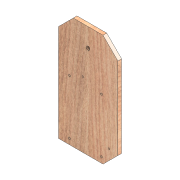
# Autodesk Inventor part: legno
Saved by Autodesk Inventor 2022 (Build 260153000, 153)
## iProperties
Created: 2025-08-06
Part Number: legno
Material: Wood (Birch)
Document SubType Name: Modeling
Designer: sacchie
Density: 0.55 g/cm^3
Appearance: Birch - Natural Polished
Author: sacchie
Autodesk Inventor part; units mm, degrees
ref_plane "YZ Plane" through (0, 0, 0) normal (1, 0, 0) x (0, 1, 0)
ref_plane "XZ Plane" through (0, 0, 0) normal (0, 1, 0) x (-1, 0, 0)
ref_plane "XY Plane" through (0, 0, 0) normal (0, 0, 1) x (1, 0, 0)
sketch "Sketch1" plane through (0, 0, 0) normal (0, 0, 1) x (1, 0, 0)
  line L0 (0, 0) -> (-160, 0)
  line L1 (-160, 0) -> (-160, 300)
  line L2 (-160, 300) -> (0, 300)
  line L3 (0, 300) -> (0, 0)
  dimension "d0" = 160
  dimension "d1" = 300
  constraints: 8 end point, 2 parallel, 1 horizontal, 1 perpendicular
  measures "d0" distance of L1.end L2.end
  measures "d1" distance of L0.end L1.end
extrude "Extrusion1" add sketch "Sketch1" along normal blind 10
sketch "Sketch2" plane through (0, 0, 10) normal (0, 0, 1) x (1, 0, 0)
  circle A0 centre (-130, 15) radius 2.55
  line L0 (-160, 0) -> (0, 0) projected
  line L1 (-160, 300) -> (-160, 0) projected
  circle A1 centre (-44, 15) radius 2.55
  circle A2 centre (-130, 161) radius 2.55
  circle A3 centre (-44, 161) radius 2.55
  circle A4 centre (-80, 250) radius 4.5984
  circle A5 centre (-50, 50) radius 5.0648 construction
  line L2 (0, 300) -> (-160, 300) projected
  line L3 (0, 0) -> (0, 300) projected
  dimension "d4" = 15
  dimension "d5" = 5.1
  dimension "d6" = 30
  dimension "d9" = 86
  dimension "d12" = 146
  dimension "d18" = 50
  dimension "d19" = 50
  dimension "d20" = 50
  dimension "d33" = 80
  constraints: 6 centre point, 1 horizontal, 1 vertical, 6 other
  measures "d4" distance from line of L0 A0.centre
  measures "d5" diameter of A0
  measures "d6" distance from line of L1 A0.centre
  measures "d9" distance of A0.centre A1.centre
  measures "d12" distance of A0.centre A2.centre
  measures "d18" distance from line of L2 A4.centre
  measures "d19" distance from line of L0 A5.centre
  measures "d20" distance from line of L3 A5.centre
  measures "d33" distance from line of L3 A4.centre
extrude "Extrusion2" cut sketch "Sketch2" against normal through all contours A0 | A1 | A2 | A3 | A4
chamfer "Chamfer1" distance 40 angle 45 3 edges at (0, 0, 5) (-160, 300, 5) (0, 300, 5)
sketch "Sketch3" plane through (0, 0, 0) normal (0, 0, -1) x (-1, 0, 0)
  line L0 (0, 300) -> (120, 300) projected
  line L1 (160, 260) -> (160, 0) projected
  line L2 (0, 0) -> (160, 300) construction
  circle A0 centre (94.1176, 176.4706) radius 2
  circle A1 centre (23.5294, 44.1176) radius 2
  line L3 (160, 0) -> (40, 0) projected
  line L4 (160, 0) -> (0, 0) construction
  line L5 (0, 260) -> (0, 0) construction
  line L6 (40, 300) -> (160, 300)
  line L7 (160, 300) -> (160, 0)
  dimension "d25" = 4
  dimension "d27" = 4
  dimension "d31" = 150
  dimension "d32" = 50
  constraints: 10 end point, 3 point on line, 2 centre point, 2 horizontal, 1 coincident, 1 perpendicular, 1 vertical
  measures "d25" diameter of A0
  measures "d27" diameter of A1
  measures "d31" distance of A1.centre A0.centre
  measures "d32" distance of L2.start A1.centre
extrude "Extrusion3" cut sketch "Sketch3" against normal blind 10
body "Solid1"
